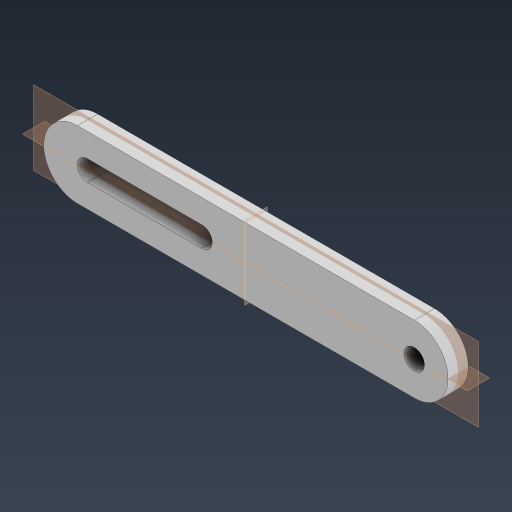
# Autodesk Inventor part: Рычаг
Saved by Autodesk Inventor 2023.2 (Build 272271030, 271C)
## iProperties
Created: 2025-12-12
Part Number: Рычаг
Material: Типовые
Document SubType Name: Modeling
Designer: Олег Коноваленко
Density: 1 g/cm^3
Appearance: По умолчанию
Author: Олег Коноваленко
Autodesk Inventor part; units mm, degrees
sketch "Эскиз1" plane through (0, 0, 0) normal (0, 0, 1) x (1, 0, 0)
  line L0 (-25, 0) -> (25, 0) construction
  line L1 (-25, -5) -> (25, -5)
  line L2 (25, 5) -> (-25, 5)
  arc A0 (-25, 5) -> (-25, -5) centre (-25, 0) ccw
  arc A1 (25, -5) -> (25, 5) centre (25, 0) ccw
  circle A2 centre (25, 0) radius 1.5
  line L3 (-25, 0) -> (-5, 0) construction
  line L4 (-23.5, -1.5) -> (-6.5, -1.5)
  line L5 (-6.5, 1.5) -> (-23.5, 1.5)
  arc A3 (-23.5, 1.5) -> (-23.5, -1.5) centre (-23.5, 0) ccw
  arc A4 (-6.5, -1.5) -> (-6.5, 1.5) centre (-6.5, 0) ccw
  point P0 (-30, 0)
  point P1 (30, 0)
  point P2 (0, 0)
  point P3 (0, 0)
  point P4 (-15, 0)
  point P5 (-5, 0)
  point P6 (-25, 0)
  dimension "d0" = 10
  dimension "d1" = 60
  dimension "d6" = 3
  dimension "d7" = 3
  dimension "d8" = 20
  constraints: 16 end point, 14 point on circle, 8 tangent, 5 centre point, 3 point on line, 2 midpoint, 2 parallel, 1 coincident, 1 concentric, 1 horizontal
  measures "d0" distance between parallel lines of L1 L2
  measures "d1" distance of point (-30, 0) point (30, 0)
  measures "d6" diameter of A2
  measures "d7" distance between parallel lines of L4 L5
  measures "d8" distance of point (-5, 0) point (-25, 0)
extrude "Выдавливание1" add sketch "Эскиз1" along normal mid plane 3
